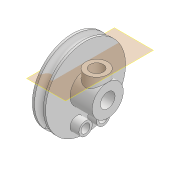
# Autodesk Inventor part: finger_pulley
Saved by Autodesk Inventor 2020.2 (Build 242310000, 310)
## iProperties
Created: 2020-04-09
Part Number: finger_pulley
Material: Generic
Document SubType Name: Modeling
Designer: Bardo91
Density: 1 g/cm^3
Appearance: Default
Author: Bardo91
Autodesk Inventor part; units mm, degrees
ref_plane "YZ Plane" through (0, 0, 0) normal (1, 0, 0) x (0, 1, 0)
ref_plane "XY Plane" through (0, 0, 0) normal (0, 0, 1) x (1, 0, 0)
sketch "Sketch1" plane through (0, 0, 0) normal (0, 0, 1) x (1, 0, 0)
  line L0 (0, 0) -> (0, 9)
  circle A0 centre (0, 9) radius 1
  line L1 (0, 9) -> (1.5, 9)
  line L2 (1.5, 9) -> (1.5, 0)
  line L3 (1.5, 0) -> (0, 0)
  line L4 (0, 0) -> (-1.5, 0)
  line L5 (-1.5, 0) -> (-1.5, 9)
  line L6 (-1.5, 9) -> (-1, 9)
  point P0 (0.5, 7.5858)
  point P1 (-0.5, 7.5858)
  point P2 (1, 9)
  point P3 (0, 8)
  dimension "d1" = 2
  dimension "d0" = 9
  dimension "d2" = 1.5
  dimension "d3" = 1.5
  constraints: 14 end point, 3 perpendicular, 3 point on line, 1 coincident, 1 horizontal, 1 vertical, 3 other
  measures "d0" distance of L0.start L0.end
  measures "d2" distance of L1.start L1.end
  measures "d3" distance of L0.start L4.end
revolve "Revolution1" add sketch "Sketch1" angle 360 about axis through (1.5, 0, 0) along (-1, 0, 0) contours L4 L5 L6 A0 L0 | L0 A0 L1 L2 L3
sketch "Sketch6" plane through (0, 0, 0) normal (0, 0, 1) x (1, 0, 0)
  line L0 (0, 0) -> (0, -6)
  circle A0 centre (0, -6) radius 1
  dimension "d14" = 6
  dimension "d15" = 2
  constraints: 2 end point, 1 centre point, 1 coincident, 1 vertical
  measures "d14" distance of L0.start L0.end
  measures "d15" diameter of A0
extrude "Extrusion4" cut sketch "Sketch6" against normal through all both and the other way through all
sketch "Sketch7" plane through (1.5, 0, 0) normal (1, 0, 0) x (0, 0, -1)
  line L0 (-6.245, -5) -> (6.245, -5) projected
  line L1 (0, -5) -> (0, -7)
  line L2 (-3.873, -7) -> (3.873, -7) projected
  line L3 (0, -6) -> (-2, -6)
  line L4 (0, -6) -> (2, -6)
  circle A0 centre (-2, -6) radius 1.5
  circle A1 centre (2, -6) radius 1.5
  point P0 (0, 0)
  dimension "d18" = 2
  dimension "d19" = 2
  dimension "d20" = 3
  dimension "d21" = 3
  constraints: 6 end point, 3 midpoint, 2 centre point, 2 coincident, 2 horizontal
  measures "d18" distance of L3.start L3.end
  measures "d19" distance of L3.start L4.end
  measures "d20" diameter of A0
  measures "d21" diameter of A1
extrude "Extrusion5" add sketch "Sketch7" along normal blind 2 contours A0 L0 | L0 A0 L2 | L2 A0 | A1 L0 | L0 A1 L2 | L2 A1
sketch "Sketch8" plane through (3.5, -6, -2) normal (1, 0, 0) x (0, 0, -1)
  circle A0 centre (0, 0) radius 1
  circle A1 centre (-4, 0) radius 1.5 projected
  circle A2 centre (-4, 0) radius 1
  point P0 (-2, 6)
  dimension "d24" = 2
  dimension "d25" = 2
  constraints: 2 centre point, 1 coincident
  measures "d24" diameter of A0
  measures "d25" diameter of A2
extrude "Extrusion6" cut sketch "Sketch8" against normal up to surface contours A0 | A2
sketch "Sketch9" plane through (1.5, 0, 0) normal (1, 0, 0) x (0, 0, -1)
  circle A0 centre (0, 0) radius 3.5
  dimension "d28" = 7
  constraints: 1 centre point, 1 coincident
  measures "d28" diameter of A0
extrude "Extrusion7" add sketch "Sketch9" along normal blind 5
sketch "Sketch10" plane through (6.5, 0, 0) normal (1, 0, 0) x (0, 0, -1)
  circle A0 centre (0, 0) radius 1.65
  dimension "d31" = 3.3
  constraints: 1 centre point, 1 coincident
  measures "d31" diameter of A0
extrude "Extrusion8" cut sketch "Sketch10" against normal through all
ref_plane "Work Plane1" through (0, 5, 0) normal (0, 1, 0) x (-1, 0, 0)
sketch "Sketch12" plane through (0, 5, 0) normal (0, 1, 0) x (-1, 0, 0)
  line L0 (-6.5, -1.65) -> (-6.5, 1.65) projected
  line L1 (-6.5, 0) -> (-1.5, 0)
  line L2 (-1.5, 9) -> (-1.5, -9) projected
  circle A0 centre (-4, 0) radius 2.5
  point P0 (0, 0)
  dimension "d36" = 5
  constraints: 3 midpoint, 2 end point, 1 centre point
  measures "d36" diameter of A0
extrude "Extrusion9" add sketch "Sketch12" against normal up to surface
sketch "Sketch13" plane through (4, 5, 0) normal (0, 1, 0) x (1, 0, 0)
  circle A0 centre (0, 0) radius 1.5
  point P0 (-4, 0)
  dimension "d39" = 3
  constraints: 1 centre point
  measures "d39" diameter of A0
extrude "Extrusion10" cut sketch "Sketch13" against normal up to surface
equation "\"d3\" = d2"
body "Solid1"
